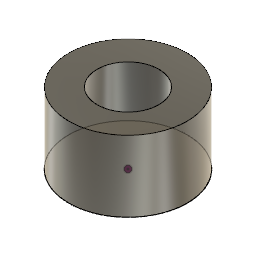
Motor Cup Stop (Autodesk Fusion 360 design; units mm, degrees)
Autodesk Fusion 360 part; units mm, degrees
sketch "Sketch1" plane through (0, 0, 0) normal (0, 0, 1) x (1, 0, 0)
  circle A0 centre (0, 0) radius 5
  dimension "d7" = 10
  constraint coincident A0.centre origin
  measures "d7" diameter of A0
extrude "Extrude2" add sketch "Sketch1" along normal blind 6 makes body 1
extrude "Extrude1" add sketch "Sketch1" along normal blind 6 separate body makes body 2
sketch "Sketch2" plane through (0, 0, 6) normal (0, 0, 1) x (-1, 0, 0)
  circle A0 centre (0, 0) radius 5
  circle A1 centre (0, 0) radius 2.6
  dimension "d12" = 5.2
  constraint coincident A0.centre A1.centre
  measures "d12" diameter of A1
extrude "Extrude3" cut sketch "Sketch2" against normal blind 106 contours A1 bodies 1 2
extrude "Extrude4" [rolled back] along distance 102.6 taper angle 0
equation "outer_radius = 5 mm"
equation "shaft_hole_radius = 2.6 mm"
equation "screw_hole_length = length"
equation "length = 6 mm"
equation "extra = 100 mm"
equation "screw_hole_width = 5 mm"
equation "d7 = outer_radius * 2"
equation "d8 = length"
equation "d10 = length"
equation "d12 = shaft_hole_radius * 2"
equation "d13 = -( length + extra )"
equation "d17 = shaft_hole_radius + extra"
